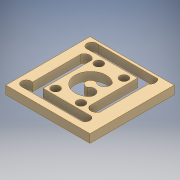
# Autodesk Inventor part: newnameC
Saved by Autodesk Inventor 2016 (Build 200138000, 138)
## iProperties
Created: 2016-10-02
Part Number: newnameC
Material: Polyethylene, High Density
Document SubType Name: Modeling
Designer: Shaan Sharma
Density: 0.952 g/cm^3
Appearance: Smooth - Off-White
Author: Shaan Sharma
Autodesk Inventor part; units mm, degrees
ref_plane "YZ Plane" through (0, 0, 0) normal (1, 0, 0) x (0, 1, 0)
ref_plane "XZ Plane" through (0, 0, 0) normal (0, 1, 0) x (-1, 0, 0)
ref_plane "XY Plane" through (0, 0, 0) normal (0, 0, 1) x (1, 0, 0)
sketch "Sketch1" plane through (0, 0, 0) normal (0, 0, 1) x (1, 0, 0)
  line L0 (44.7404, -16.6127) -> (-43.4425, -16.6127)
  arc A0 (44.7404, -16.6127) -> (46.8806, -2.4194) centre (44.7404, -9.3547) ccw
  arc A1 (-41.9354, -2.4194) -> (-43.4425, -16.6127) centre (-44.2086, -9.3547) ccw
  line L1 (48.387, 82.2579) -> (48.387, 9.6774)
  arc A2 (-25.6909, 70.9206) -> (-41.9354, 70.9676) centre (-33.8226, 67.6679) ccw
  line L2 (-41.9354, -2.4194) -> (-41.9354, 70.9676)
  line L3 (-25.6909, -2.4194) -> (-25.6909, 70.9206)
  line L4 (-25.6909, -2.4194) -> (46.8806, -2.4194)
  line L5 (-57.912, 100.584) -> (69.088, 100.584)
  line L6 (69.088, 100.584) -> (69.088, -26.416)
  line L7 (69.088, -26.416) -> (-57.912, -26.416)
  line L8 (-57.912, -26.416) -> (-57.912, 100.584)
  arc A3 (32.258, 9.6774) -> (48.387, 9.6774) centre (40.3225, 12.3185) ccw
  arc A4 (48.387, 82.2579) -> (48.387, 96.774) centre (42.691, 89.5159) ccw
  line L9 (32.258, 82.2579) -> (-41.9354, 82.2579)
  line L10 (48.387, 96.774) -> (-41.9354, 96.774)
  line L11 (32.258, 9.6774) -> (32.258, 82.2579)
  arc A5 (-41.9354, 96.774) -> (-41.9354, 82.2579) centre (-43.9372, 89.5159) ccw
  point P0 (0, 0)
  dimension "d0" = 127
  dimension "d1" = 127
  constraints: 24 end point, 12 point on circle, 6 centre point, 4 horizontal, 3 vertical, 2 parallel, 1 perpendicular, 1 tangent
  measures "d0" distance of L5.end L6.end
  measures "d1" distance of L6.end L7.end
extrude "Extrusion1" add sketch "Sketch1" along normal blind 12.7
sketch "Sketch2" plane through (0, 0, 12.7) normal (0, 0, 1) x (1, 0, 0)
  circle A0 centre (22, 7) radius 6.35
  circle A1 centre (-16, 6.6796) radius 6.35
  circle A2 centre (-16, 72) radius 6.35
  circle A3 centre (22, 72) radius 6.35
  point P0 (0, 0)
  dimension "d4" = 12.7
  dimension "d5" = 12.7
  dimension "d6" = 12.7
  dimension "d7" = 12.7
  constraints: 4 centre point
  measures "d4" diameter of A0
  measures "d5" diameter of A1
  measures "d6" diameter of A2
  measures "d7" diameter of A3
hole "Hole1" at (-16, 6.6796, 12.7) at (22, 72, 12.7) at (-16, 72, 12.7) at (22, 7, 12.7) direction (0, 0, -1) diameter 12.7 end through all
sketch "Sketch3" plane through (0, 0, 12.7) normal (0, 0, 1) x (1, 0, 0)
  arc A0 (20.8111, 55.9606) -> (21.1932, 22.4134) centre (4.585, 39) ccw
  arc A1 (8, 45) -> (8.4788, 33.299) centre (4.585, 39) ccw
  arc A2 (6.7211, 45.565) -> (19.6498, 57) centre (12.644, 51.8946) ccw
  arc A3 (18.8086, 20.3282) -> (5.9993, 32.2426) centre (13.4301, 27.3887) ccw
  circle A4 centre (-16, 72) radius 6.35 projected
  circle A5 centre (-16, 6.6796) radius 6.35 projected
  circle A6 centre (22, 72) radius 6.35 projected
  circle A7 centre (22, 7) radius 6.35 projected
  arc A8 (48.387, 82.2579) -> (48.387, 96.774) centre (42.691, 89.5159) ccw projected
  line L0 (48.387, 82.2579) -> (48.387, 9.6774) projected
  arc A9 (32.258, 9.6774) -> (48.387, 9.6774) centre (40.3225, 12.3185) ccw projected
  line L1 (32.258, 9.6774) -> (32.258, 82.2579) projected
  line L2 (32.258, 82.2579) -> (-41.9354, 82.2579) projected
  arc A10 (-41.9354, 96.774) -> (-41.9354, 82.2579) centre (-43.9372, 89.5159) ccw projected
  line L3 (-41.9354, 96.774) -> (48.387, 96.774) projected
  arc A11 (-41.9354, -2.4194) -> (-43.4425, -16.6127) centre (-44.2086, -9.3547) ccw projected
  line L4 (-41.9354, -2.4194) -> (-41.9354, 70.9676) projected
  arc A12 (-25.6909, 70.9206) -> (-41.9354, 70.9676) centre (-33.8226, 67.6679) ccw projected
  line L5 (-25.6909, 70.9206) -> (-25.6909, -2.4194) projected
  line L6 (-25.6909, -2.4194) -> (46.8806, -2.4194) projected
  arc A13 (44.7404, -16.6127) -> (46.8806, -2.4194) centre (44.7404, -9.3547) ccw projected
  line L7 (44.7404, -16.6127) -> (-43.4425, -16.6127) projected
  line L8 (69.088, 100.584) -> (-57.912, 100.584) projected
  line L9 (-57.912, 100.584) -> (-57.912, -26.416) projected
  line L10 (-57.912, -26.416) -> (69.088, -26.416) projected
  line L11 (69.088, -26.416) -> (69.088, 100.584) projected
  point P0 (0, 0)
  point P1 (20.2164, 21.4898)
  point P2 (20.9887, 55.7889)
  constraints: 14 point on circle, 4 centre point, 1 coincident, 1 tangent
emboss "Emboss1" sketch "Sketch3" operation cut depth 12.7 direction (0, 0, -1) contours A2 A1 A3 A0
body "Solid1"
